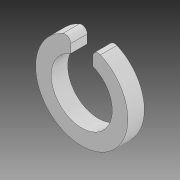
# Autodesk Inventor part: 2002_Rx_Tx Coil Spacer_Glass_v3
Saved by Autodesk Inventor 2021 (Build 250183000, 183)
## iProperties
Created: 2022-08-09
Part Number: 2002_Rx_Tx Coil Spacer_Glass_v3
Material: Generic
Document SubType Name: Modeling
Designer: Eli
Density: 1 g/cm^3
Appearance: Default
Author: Eli
Autodesk Inventor part; units mm, degrees
ref_plane "YZ Plane" through (0, 0, 0) normal (1, 0, 0) x (0, 1, 0)
ref_plane "XZ Plane" through (0, 0, 0) normal (0, 1, 0) x (-1, 0, 0)
ref_plane "XY Plane" through (0, 0, 0) normal (0, 0, 1) x (1, 0, 0)
sketch "Sketch1" plane through (0, 0, 0) normal (0, 0, 1) x (1, 0, 0)
  circle A0 centre (0, 0) radius 5.55
  circle A1 centre (0, 0) radius 8.375
  line L0 (-2, 8.375) -> (2, 8.375)
  line L1 (2, 8.375) -> (2, 0)
  line L2 (2, 0) -> (-2, 0)
  line L3 (-2, 0) -> (-2, 8.375)
  point P0 (-2, 5.1771)
  point P1 (-2, 8.1327)
  point P2 (2, 8.1327)
  point P3 (2, 5.1771)
  dimension "d0" = 11.1
  dimension "d1" = 16.75
  dimension "d2" = 4
  constraints: 8 end point, 3 coincident, 2 centre point, 2 parallel, 1 horizontal, 1 midpoint, 1 perpendicular, 1 tangent
  measures "d0" diameter of A0
  measures "d1" diameter of A1
  measures "d2" distance of L0.start L0.end
extrude "Extrusion1" add sketch "Sketch1" along normal blind 3 contours A0 L1 A1 L3 picked at (7.294, -1.1285)
fillet "Fillet1" radius 1 2 edges at (-2, 8.1327, 1.5) (2, 8.1327, 1.5)
body "Solid1"
